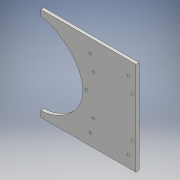
# Autodesk Inventor part: BaseSuperior
Saved by Autodesk Inventor 2017 SP1 (Build 210196100, 196)
## iProperties
Part Number: BaseSuperior
Material: Genérico
Document SubType Name: Modeling
Designer: Juan
Density: 1 g/cm^3
Appearance: Valor por defecto
Author: Juan
Autodesk Inventor part; units mm, degrees
ref_plane "YZ Plane" through (0, 0, 0) normal (1, 0, 0) x (0, 1, 0)
ref_plane "XZ Plane" through (0, 0, 0) normal (0, 1, 0) x (-1, 0, 0)
sketch "Boceto1" plane through (0, 0, 0) normal (0, 1, 0) x (-1, 0, 0)
  line L0 (125, 0) -> (0, 0)
  line L1 (0, 0) -> (0, 123)
  line L2 (0, 123) -> (125, 123)
  line L3 (125, 123) -> (125, 115)
  line L4 (125, 0) -> (125, 8)
  line L5 (125, 115) -> (96.7331, 115) construction
  line L6 (96.7331, 115) -> (18.5523, 55.1972) construction
  line L7 (18.5523, 55.1972) -> (92.1923, 8) construction
  line L8 (92.1923, 8) -> (125, 8) construction
  spline S0 degree 4 poles (125, 115) (96.7331, 115) (18.5523, 55.1972) (92.1923, 8) (125, 8) knots 1 1 1 1 1 2 2 2 2 2
  dimension "d0" = 125
  dimension "d1" = 123
  dimension "d2" = 125
  dimension "d3" = 8
  dimension "d4" = 8
  dimension "d5" = 52.587
  dimension "d6" = 57.343
  dimension "d7" = 32.5699
  dimension "d8" = 56.4825
  constraints: 10 end point, 3 horizontal, 3 vertical, 1 coincident, 1 perpendicular, 3 other
  measures "d0" distance of L0.start L0.end
  measures "d1" distance of L0.end L1.end
  measures "d2" distance of L1.end L2.end
  measures "d3" distance of L2.end L3.end
  measures "d4" distance of L0.start L4.end
  measures "d5" angle of L6 L3
  measures "d6" angle of L3 L7
  measures "d7" distance from line of point (0, 0) L6
  measures "d8" distance from line of point (0, 0) L7
extrude "Extrusión1" add sketch "Boceto1" along normal blind 4
sketch "Boceto2" plane through (0, 4, 0) normal (0, 1, 0) x (1, 0, 0)
  point P0 (0, 0)
sketch "Boceto3" plane through (0, 4, 0) normal (0, 1, 0) x (1, 0, 0)
  line L0 (-125, -123) -> (0, -123) construction
  line L1 (0, -123) -> (-10, -123) construction
  line L2 (-10, -123) -> (-10, -108.009) construction
  line L3 (0, 0) -> (-125, 0) construction
  line L4 (0, 0) -> (-10, 0) construction
  line L5 (-10, 0) -> (-10, -14.991) construction
  dimension "d12" = 10
  dimension "d13" = 14.991
  dimension "d14" = 10
  dimension "d15" = 14.991
  constraints: 8 end point, 2 perpendicular, 2 point on line
  measures "d12" distance of L0.end L1.end
  measures "d13" distance of L1.end L2.end
  measures "d14" distance of L3.start L4.end
  measures "d15" distance of L4.end L5.end
sketch "Boceto4" plane through (0, 4, 0) normal (0, 1, 0) x (1, 0, 0)
  point P0 (0, 0)
sketch "Boceto5" plane through (0, 4, 0) normal (0, 1, 0) x (1, 0, 0)
  point P0 (0, 0)
hole "Agujero3" at (-10, 4, 105.0128) direction (0, -1, 0) diameter 3 end through all
sketch "Boceto6" plane through (0, 4, 0) normal (0, 1, 0) x (1, 0, 0)
  point P0 (0, 0)
hole "Agujero4" at (-10.0142, 4, 14.9403) direction (0, -1, 0) diameter 3 end through all
sketch "Boceto7" plane through (0, 4, 0) normal (0, 1, 0) x (1, 0, 0)
  circle A0 centre (-10, -105.0128) radius 1.5 construction
  line L0 (-10, -105.0128) -> (-60, -105.0128) construction
  circle A1 centre (-10.0142, -14.9403) radius 1.5 construction
  line L1 (-10.0142, -14.9403) -> (-60.0142, -14.9403) construction
  point P0 (0, 0)
  dimension "d50" = 50
  dimension "d51" = 50
  constraints: 4 end point, 2 horizontal
  measures "d50" distance of L0.start L0.end
  measures "d51" distance of L1.start L1.end
hole "Agujero5" at (-59.9814, 4, 105.0154) direction (0, -1, 0) diameter 3 end through all
hole "Agujero6" at (-60.0068, 4, 14.9437) direction (0, -1, 0) diameter 3 end through all
sketch "Boceto8" plane through (0, 4, 0) normal (0, 1, 0) x (1, 0, 0)
  line L0 (0, -105.0128) -> (-5, -105.0128) construction
  line L1 (0, 0) -> (0, -123) construction
  line L2 (0, -14.7274) -> (-5, -14.7274) construction
  line L3 (-5, -105.0128) -> (-5, -120) construction
  line L4 (-5, -120) -> (-5, -86.5) construction
  line L5 (-4.9612, -0.0001) -> (-4.9612, -33.5001) construction
  dimension "d70" = 5
  dimension "d72" = 5
  dimension "d74" = 33.5
  dimension "d76" = 33.5
  constraints: 10 end point, 2 point on line, 2 vertical, 1 horizontal, 1 perpendicular
  measures "d70" distance of L0.start L0.end
  measures "d72" distance of L2.start L2.end
  measures "d74" distance of L3.end L4.end
  measures "d76" distance of L5.start L5.end
hole "Agujero7" at (-5, 4, 86.5014) direction (0, -1, 0) diameter 3 end through all
hole "Agujero8" at (-4.9615, 4, 33.4984) direction (0, -1, 0) diameter 3 end through all
sketch "Boceto9" plane through (0, 4, 0) normal (0, 1, 0) x (1, 0, 0)
  circle A0 centre (-4.9615, -33.4984) radius 1.5 construction
  line L0 (-4.9615, -33.4984) -> (-55.4625, -33.4984) construction
  circle A1 centre (-5, -86.5014) radius 1.5 construction
  line L1 (-5, -86.5014) -> (-5, -123) construction
  line L2 (-125, -123) -> (0, -123) construction
  line L3 (-5, -86.5014) -> (-55.501, -86.5014) construction
  point P0 (0, 0)
  dimension "d95" = 50.501
  dimension "d98" = 50.501
  constraints: 6 end point, 2 horizontal, 1 point on line, 1 vertical
  measures "d95" distance of L0.start L0.end
  measures "d98" distance of L1.start L3.end
hole "Agujero9" at (-55.4892, 4, 86.5021) direction (0, -1, 0) diameter 3 end through all
hole "Agujero10" at (-55.5221, 4, 33.5513) direction (0, -1, 0) diameter 3 end through all
sketch "Boceto10" plane through (0, 4, 0) normal (0, 1, 0) x (1, 0, 0)
  point P0 (0, 0)
ref_plane "Plano de trabajo2" through (0, 4, 0) normal (0, 1, 0) x (1, 0, 0)
sketch "Boceto11" plane through (0, 4, 0) normal (0, 1, 0) x (1, 0, 0)
  line L0 (0, 0) -> (-125, 0) construction
  line L1 (0, 0) -> (0, -61.5) construction
  line L2 (0, -123) -> (0, 0) construction
  line L3 (0, -61.5) -> (-70.0164, -61.5) construction
  line L4 (-70.0164, -61.5) -> (-65.0164, -61.5) construction
  dimension "d118" = 5
  constraints: 6 end point, 1 horizontal, 1 midpoint, 1 point on line
  measures "d118" distance of L3.end L4.end
hole "Agujero11" at (-65.0164, 4, 61.5) direction (0, -1, 0) diameter 3 end through all
